Autodesk Inventor part; units mm, degrees
(part 4 of 4)
  line L457 (51.9809, 24.7439) -> (52.0774, 24.7439) projected
  line L458 (53.47, 25.2204) -> (53.47, 25.2686) projected
  line L459 (53.4643, 27.4866) -> (53.4955, 27.6029) projected
  line L460 (53.4955, 27.6029) -> (54.2925, 27.6029) projected
  line L461 (57.3217, 27.6029) -> (57.3217, 25.2657) projected
  line L462 (55.0101, 24.7439) -> (55.1065, 24.7439) projected
  line L463 (56.4992, 25.2204) -> (56.4992, 25.2686) projected
  line L464 (56.4935, 27.4866) -> (56.5247, 27.6029) projected
  line L465 (56.5247, 27.6029) -> (57.3217, 27.6029) projected
  line L466 (58.4307, 26.7406) -> (58.4307, 26.7548) projected
  line L467 (59.8772, 26.8683) -> (59.8772, 26.8569) projected
  line L468 (72.5895, 26.0174) -> (72.6689, 26.0174) projected
  line L469 (72.6689, 26.0174) -> (72.6689, 25.1948) projected
  line L470 (80.4432, 24.9623) -> (80.4432, 27.6029) projected
  line L471 (80.4432, 27.6029) -> (81.2658, 27.6029) projected
  line L472 (81.2658, 27.6029) -> (81.2658, 27.2228) projected
  line L473 (91.0085, 26.423) -> (91.0085, 26.1251) projected
  line L474 (91.0085, 26.1251) -> (89.2017, 26.1251) projected
  line L475 (91.4793, 25.7961) -> (91.4793, 27.0299) projected
  line L476 (91.4793, 27.0299) -> (91.1645, 27.0299) projected
  line L477 (91.1645, 27.0299) -> (91.1645, 27.6029) projected
  line L478 (91.1645, 27.6029) -> (91.4793, 27.6029) projected
  line L479 (91.4793, 27.6029) -> (91.4793, 28.3573) projected
  line L480 (91.4793, 28.3573) -> (92.3018, 28.3573) projected
  line L481 (92.3018, 28.3573) -> (92.3018, 27.6029) projected
  line L482 (92.3018, 27.6029) -> (93.096, 27.6029) projected
  line L483 (93.096, 27.6029) -> (93.096, 27.0299) projected
  line L484 (93.096, 27.0299) -> (92.3018, 27.0299) projected
  line L485 (92.3018, 27.0299) -> (92.3018, 26.0911) projected
  line L486 (27.7761, 19.5133) -> (27.7761, 18.5968) projected
  line L487 (41.7358, 17.5096) -> (41.7358, 17.1778) projected
  line L488 (41.7358, 17.1778) -> (39.7226, 17.1778) projected
  line L489 (41.5841, 16.8048) -> (41.6821, 16.8048) projected
  line L490 (58.8939, 15.882) -> (58.8939, 16.1949) projected
  line L491 (58.9003, 17.813) -> (58.9003, 17.8288) projected
  line L492 (57.3769, 18.05) -> (57.2979, 18.05) projected
  line L493 (57.2979, 18.05) -> (57.2979, 18.7611) projected
  line L494 (59.8041, 17.8825) -> (59.8041, 15.882) projected
  line L495 (59.8041, 15.882) -> (58.8939, 15.882) projected
  line L496 (73.9535, 17.813) -> (73.9535, 17.8288) projected
  line L497 (72.4302, 18.05) -> (72.3511, 18.05) projected
  line L498 (56.5983, 11.0629) -> (56.5983, 10.731) projected
  line L499 (56.5983, 10.731) -> (54.5851, 10.731) projected
  line L500 (56.4466, 10.3581) -> (56.5446, 10.3581) projected
  line L501 (84.9286, 11.0629) -> (84.9286, 10.731) projected
  line L502 (84.9286, 10.731) -> (82.9154, 10.731) projected
  point P0 (0, 0)
  point P1 (47.4432, 3.0913)
  point P2 (46.2833, 2.5793)
  point P3 (47.7845, 4.6114)
  point P4 (88.9329, 11.8119)
  point P5 (88.5252, 11.6286)
  point P6 (88.3514, 10.8985)
  point P7 (84.4135, 9.4415)
  point P8 (83.7213, 9.3562)
  point P9 (74.6097, 11.8814)
  point P10 (65.0778, 11.7676)
  point P11 (64.4173, 10.8922)
  point P12 (58.8327, 11.5085)
  point P13 (58.4566, 11.6949)
  point P14 (58.8959, 12.4566)
  point P15 (59.822, 11.3505)
  point P16 (59.822, 9.4352)
  point P17 (56.5446, 9.5996)
  point P18 (56.0831, 9.4415)
  point P19 (55.391, 9.3562)
  point P20 (52.3633, 10.6457)
  point P21 (52.0725, 11.0881)
  point P22 (51.412, 11.1292)
  point P23 (51.2318, 11.1292)
  point P24 (51.2856, 10.1463)
  point P25 (52.1073, 10.2222)
  point P26 (46.2225, 11.6286)
  point P27 (46.0487, 10.8985)
  point P28 (46.6302, 11.8119)
  point P29 (39.456, 13.8251)
  point P30 (38.669, 12.7948)
  point P31 (36.6906, 13.509)
  point P32 (36.6906, 9.4352)
  point P33 (35.7741, 13.509)
  point P34 (30.3602, 10.4655)
  point P35 (30.3602, 9.4352)
  point P36 (29.4342, 10.4655)
  point P37 (25.0159, 12.4787)
  point P38 (20.7271, 10.4655)
  point P39 (20.7271, 9.4352)
  point P40 (15.3165, 11.6286)
  point P41 (15.1426, 10.8985)
  point P42 (73.5774, 15.9262)
  point P43 (73.0117, 15.803)
  point P44 (72.3511, 18.7611)
  point P45 (73.4036, 18.9065)
  point P46 (71.6242, 18.8244)
  point P47 (71.6242, 15.882)
  point P48 (70.7077, 18.8244)
  point P49 (66.1314, 17.1525)
  point P50 (66.3178, 16.4414)
  point P51 (63.0815, 17.5602)
  point P52 (63.0815, 15.882)
  point P53 (64.7186, 19.0393)
  point P54 (63.0815, 19.0393)
  point P55 (58.5242, 15.9262)
  point P56 (57.9584, 15.803)
  point P57 (53.0344, 18.0279)
  point P58 (53.3979, 17.7561)
  point P59 (53.9636, 17.6265)
  point P60 (54.6084, 16.8017)
  point P61 (54.2354, 16.0937)
  point P62 (53.1798, 15.803)
  point P63 (54.0584, 18.1543)
  point P64 (53.5085, 18.2744)
  point P65 (51.7987, 17.3516)
  point P66 (50.2817, 15.7903)
  point P67 (48.7615, 17.3516)
  point P68 (50.2817, 18.916)
  point P69 (41.2207, 15.8883)
  point P70 (40.5285, 15.803)
  point P71 (27.7919, 16.1032)
  point P72 (26.3191, 15.7998)
  point P73 (25.6554, 18.8117)
  point P74 (25.3204, 17.8509)
  point P75 (26.5973, 16.5172)
  point P76 (26.8438, 16.5267)
  point P77 (26.8438, 17.2947)
  point P78 (26.0884, 17.2947)
  point P79 (96.6896, 27.6851)
  point P80 (98.051, 26.2811)
  point P81 (96.6896, 24.88)
  point P82 (92.7017, 25.4841)
  point P83 (93.096, 24.985)
  point P84 (92.4408, 24.9112)
  point P85 (90.8723, 25.7905)
  point P86 (90.9603, 25.7905)
  point P87 (90.9603, 25.1097)
  point P88 (90.5462, 24.9679)
  point P89 (89.925, 24.8914)
  point P90 (83.3788, 28.6211)
  point P91 (83.3788, 27.9801)
  point P92 (82.5081, 27.9801)
  point P93 (82.5081, 28.6211)
  point P94 (81.8132, 26.8569)
  point P95 (78.645, 27.6851)
  point P96 (80.0064, 26.2811)
  point P97 (78.645, 24.88)
  point P98 (74.1693, 25.4643)
  point P99 (74.5948, 25.6515)
  point P100 (74.5948, 26.1989)
  point P101 (74.002, 26.1025)
  point P102 (70.9757, 27.6057)
  point P103 (70.6778, 26.7066)
  point P104 (71.6252, 27.8751)
  point P105 (62.7532, 25.8982)
  point P106 (62.3675, 26.3691)
  point P107 (61.942, 26.5421)
  point P108 (59.1738, 27.9461)
  point P109 (58.7455, 27.6114)
  point P110 (59.6106, 27.5546)
  point P111 (60.1892, 25.1807)
  point P112 (59.1653, 24.88)
  point P113 (60.5551, 25.9351)
  point P114 (56.9274, 24.2447)
  point P115 (55.9205, 23.9696)
  point P116 (55.0101, 24.083)
  point P117 (52.8914, 23.9696)
  point P118 (51.9809, 24.083)
  point P119 (54.2925, 25.2657)
  point P120 (53.8983, 24.2447)
  point P121 (45.7325, 26.9902)
  point P122 (42.7289, 27.6851)
  point P123 (44.0903, 26.2811)
  point P124 (42.7289, 24.88)
  point P125 (38.3667, 25.8869)
  point P126 (38.3667, 24.9623)
  point P127 (35.2978, 25.0927)
  point P128 (35.2637, 24.9623)
  point P129 (35.9501, 24.9112)
  point P130 (25.7111, 28.6211)
  point P131 (25.7111, 27.9801)
  point P132 (24.8403, 28.6211)
  point P133 (23.0818, 27.0555)
  point P134 (22.489, 26.3294)
  point P135 (22.991, 25.6486)
  point P136 (20.41, 28.6183)
  point P137 (15.5089, 27.6029)
  point P138 (15.5089, 26.6782)
  point P139 (13.0555, 26.6442)
  point P140 (13.5632, 26.5279)
  point P141 (14.1418, 25.7876)
  point P142 (13.8071, 25.1523)
  point P143 (12.8598, 24.8914)
  point P144 (13.1235, 27.6738)
  point P145 (13.9603, 26.8172)
  point P146 (13.6483, 27.0016)
  point P147 (13.1547, 27.1093)
  point P148 (12.7293, 26.8881)
  point P149 (69.63, 34.3142)
  point P150 (69.3001, 35.2947)
  point P151 (69.9821, 35.4998)
  point P152 (57.5826, 33.4094)
  point P153 (57.5068, 34.2696)
  point P154 (57.0076, 34.5237)
  point P155 (55.0242, 34.2696)
  point P156 (54.525, 34.5237)
  point P157 (53.9189, 35.0273)
  point P158 (55.1535, 35.5978)
  point P159 (56.2633, 34.8758)
  point P160 (57.6316, 35.5978)
  point P161 (58.5364, 35.2279)
  point P162 (37.3565, 31.3993)
  point P163 (36.5586, 31.2254)
  point P164 (35.9971, 33.7214)
  point P165 (37.8869, 34.0601)
  point P166 (37.8869, 34.0824)
  point P167 (36.8706, 34.6886)
  point P168 (35.6271, 35.3972)
  point P169 (37.1113, 35.6023)
  point P170 (32.1907, 35.4908)
  point P171 (31.7227, 34.078)
  point P172 (33.2203, 32.2595)
  point P173 (34.1563, 32.5536)
  point P174 (34.0894, 31.3904)
  point P175 (32.9886, 31.2299)
  point P176 (30.2965, 34.0824)
  point P177 (32.993, 36.9438)
  point P178 (34.085, 36.8057)
  point P179 (34.8516, 36.4848)
  point P180 (34.8516, 35.1744)
  point P181 (34.7134, 35.1744)
  point P182 (34.1162, 35.629)
  point P183 (33.2114, 35.9143)
  point P184 (46.382, 33.4094)
  point P185 (44.2426, 31.2076)
  point P186 (42.0988, 33.4094)
  point P187 (44.2426, 35.6156)
  point P188 (49.2211, 34.3142)
  point P189 (48.8913, 35.2947)
  point P190 (49.5732, 35.4998)
  point P191 (62.9444, 31.3458)
  point P192 (61.9683, 31.2254)
  point P193 (59.5392, 33.3871)
  point P194 (61.7588, 35.6156)
  point P195 (63.6709, 33.6322)
  point P196 (61.2284, 32.3754)
  point P197 (62.102, 32.1614)
  point P198 (62.9444, 32.3442)
  point P199 (65.9217, 31.2566)
  constraints: 74 vertical alignment, 60 horizontal alignment, 16 end point, 16 point on circle, 8 centre point, 378 other
sketch "Esboço5" plane through (2, 0, 0) normal (1, 0, 0) x (0, 0, -1)
  point P0 (0, 0)
extrude "Extrusão4" add sketch "Esboço4" along normal blind 0.5 contours L333 A9 L332 A8 L331 A7 L330 A6 L329 A5 L328 A4 L327 A3 L326 A2
equation "\"d4\" = d5"
equation "\"d6\" = d7"
equation "\"d11\" = 0.5 * d10"
equation "\"d12\" = d11"
